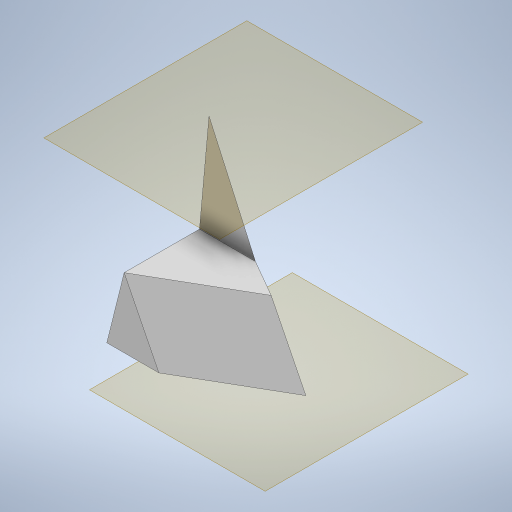
# Autodesk Inventor part: Деталь2
Saved by Autodesk Inventor 2023.2 (Build 272271030, 271C)
## iProperties
Created: 2023-09-29
Part Number: Деталь2
Material: Типовые
Document SubType Name: Modeling
Designer: User
Density: 1 g/cm^3
Appearance: По умолчанию
Author: User
Autodesk Inventor part; units mm, degrees
ref_plane "YZ Plane" through (0, 0, 0) normal (1, 0, 0) x (0, 1, 0)
ref_plane "XZ Plane" through (0, 0, 0) normal (0, 1, 0) x (-1, 0, 0)
ref_plane "XY Plane" through (0, 0, 0) normal (0, 0, 1) x (1, 0, 0)
sketch "Эскиз1" plane through (0, 0, 0) normal (0, 1, 0) x (-1, 0, 0)
  line L0 (-24.9696, 12.6351) -> (42.5304, 51.6062)
  line L1 (42.5304, 51.6062) -> (42.5304, -26.3361)
  line L2 (42.5304, -26.3361) -> (-24.9696, 12.6351)
  point P0 (0, 0)
  point P1 (20.0304, 12.6351)
  constraints: 6 end point, 7 other
ref_plane "РабПлоскость2" through (0, 90, 0) normal (0, 1, 0) x (-1, 0, 0)
ref_plane "РабПлоскость1" through (0, 0, 0) normal (0, 1, 0) x (-1, 0, 0)
sketch "Эскиз3" plane through (0, 90, 0) normal (0, 1, 0) x (-1, 0, 0)
  point P0 (0, 0)
  point P1 (20.0304, 12.635)
loft "Лофт1" add profiles "Эскиз1" section 2 point at (-20.0304, 90, 12.635)
sketch "Эскиз4" plane through (0, 0, 0) normal (1, 0, 0) x (0, 1, 0)
  line L0 (0, 51.6062) -> (90, 12.635) projected
  line L1 (32.265, 37.6351) -> (32.265, 12.6351)
  line L2 (0, 12.6351) -> (90, 12.635) projected
  line L3 (32.265, 12.6351) -> (32.265, 2.6351)
  line L4 (0, -26.3361) -> (90, 12.635) projected
  line L5 (32.265, 2.6351) -> (90, 12.635)
  point P0 (0, 0)
  dimension "d6" = 25
  dimension "d7" = 10
  constraints: 6 end point, 2 point on line, 2 vertical
  measures "d6" distance of L1.start L1.end
  measures "d7" distance of L1.end L3.end
extrude "Выдавливание1" cut sketch "Эскиз4" along normal mid plane 1000
sketch "Эскиз5" plane through (0, 0, 0) normal (1, 0, 0) x (0, 1, 0)
  line L0 (0, 51.6062) -> (32.265, 37.6351) projected
  line L1 (32.265, 37.6351) -> (0, 37.6351)
  line L2 (0, 51.6062) -> (0, -26.3361) projected
  point P0 (0, 0)
  constraints: 2 end point, 1 horizontal, 1 point on line
extrude "Выдавливание2" cut sketch "Эскиз5" along normal mid plane 100
